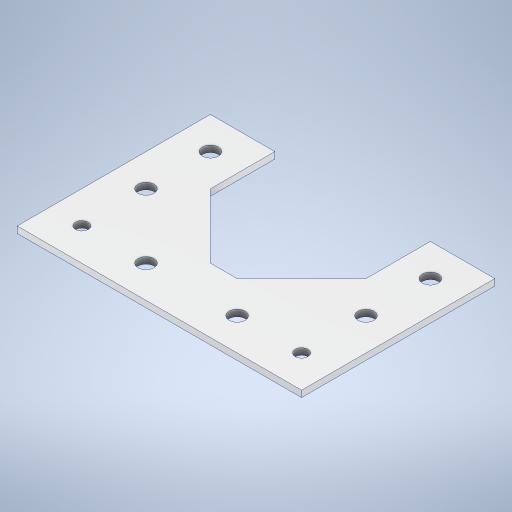
# Autodesk Inventor part: Connect_u2020
Saved by Autodesk Inventor 2024 (Build 280153000, 153)
## iProperties
Created: 2025-12-19
Part Number: Connect_u2020
Material: Aluminum 6061
Document SubType Name: Modeling
Designer: schar
Density: 2.7 g/cm^3
Appearance: Aluminum - Flat
Description: U-Connector 2020 Profile
Author: schar
Autodesk Inventor part; units mm, degrees
ref_plane "YZ Plane" through (0, 0, 0) normal (1, 0, 0) x (0, 1, 0)
ref_plane "XZ Plane" through (0, 0, 0) normal (0, 1, 0) x (-1, 0, 0)
ref_plane "XY Plane" through (0, 0, 0) normal (0, 0, 1) x (1, 0, 0)
sketch "Sketch2" plane through (0, 0, 0) normal (0, 1, 0) x (-1, 0, 0)
  line L0 (0, 0) -> (88.3, 0)
  line L1 (88.3, 0) -> (88.3, -60)
  line L2 (88.3, -60) -> (0, -60)
  line L3 (0, -60) -> (0, 0)
  line L4 (88.3, -60) -> (68.3, -60)
  line L5 (68.3, 0) -> (68.3, -20)
  line L6 (0, -60) -> (20, -60)
  line L7 (20, 0) -> (20, -20)
  line L8 (20, -20) -> (20, -60)
  line L9 (20, -20) -> (68.3, -20)
  line L10 (68.3, -20) -> (68.3, -60)
  line L11 (68.3, -20) -> (48.3, -20)
  line L12 (48.3, -20) -> (68.3, -40)
  line L13 (20, -20) -> (40, -20)
  line L14 (40, -20) -> (20, -40)
  line L15 (78.3, -60) -> (78.3, -40)
  line L16 (78.3, -40) -> (78.3, -50)
  line L17 (78.3, -40) -> (78.3, -50)
  line L18 (78.3, -40) -> (78.3, -30)
  circle A0 centre (78.3, -30) radius 2.5
  circle A1 centre (78.3, -50) radius 2.5
  line L19 (44.15, -60) -> (44.15, -44.15)
  circle A2 centre (10, -30) radius 2.5
  circle A3 centre (10, -50) radius 2.5
  line L20 (44.15, -20) -> (44.15, -10)
  line L21 (44.15, -10) -> (58.3, -10)
  line L22 (44.15, -10) -> (30, -10)
  circle A4 centre (58.3, -10) radius 2.5
  circle A5 centre (30, -10) radius 2.5
  dimension "d0" = 88.3
  dimension "d1" = 60
  dimension "d2" = 20
  dimension "d3" = 20
  dimension "d4" = 20
  dimension "d5" = 20
  dimension "d6" = 20
  dimension "d7" = 20
  dimension "d9" = 20
  dimension "d10" = 5
  dimension "d11" = 5
  dimension "d12" = 5
  dimension "d13" = 5
  constraints: 46 end point, 6 centre point, 6 point on line, 6 vertical, 5 midpoint, 4 coincident, 3 horizontal, 3 perpendicular, 2 parallel, 2 symmetric about line, 1 collinear, 2 other
  measures "d0" distance of L1.end L2.end
  measures "d1" distance of L0.end L1.end
  measures "d2" distance of L1.end L4.end
  measures "d3" distance of L5.start L5.end
  measures "d4" distance of L2.end L6.end
  measures "d5" distance of L7.start L7.end
  measures "d6" distance of L5.end L11.end
  measures "d7" distance of L7.end L13.end
  measures "d9" distance of L15.start L15.end
  measures "d10" diameter of A0
  measures "d11" diameter of A1
  measures "d12" diameter of A4
  measures "d13" diameter of A5
extrude "Extrusion1" add sketch "Sketch2" along normal blind 2 contours L0 L7 L8 L2 L3 | L0 L5 L9 L7 | L0 L1 L2 L10 L5 | L9 L14 L8 | L10 L12 L9
sketch "Sketch3" plane through (0, 2, 0) normal (0, 1, 0) x (1, 0, 0)
  line L0 (0, 0) -> (0, 10)
  line L1 (0, 0) -> (0, 60) projected
  line L2 (0, 10) -> (-10, 10)
  line L3 (-88.2278, 0) -> (-88.3, 9.9997)
  line L4 (-88.3, 60) -> (-88.3, 0) projected
  line L5 (-88.3, 9.9997) -> (-78.3003, 10.072)
  circle A0 centre (-78.3003, 10.072) radius 2
  circle A1 centre (-10, 10) radius 2
  dimension "d16" = 10
  dimension "d17" = 10
  dimension "d18" = 10
  dimension "d19" = 10
  dimension "d20" = 4
  dimension "d21" = 4
  constraints: 8 end point, 2 centre point, 2 coincident, 2 perpendicular, 2 point on line
  measures "d16" distance of L0.start L0.end
  measures "d17" distance of L0.end L2.end
  measures "d18" distance of L3.start L3.end
  measures "d19" distance of L3.end L5.end
  measures "d20" diameter of A0
  measures "d21" diameter of A1
extrude "Extrusion2" cut sketch "Sketch3" against normal blind 2
body "Solid1"
